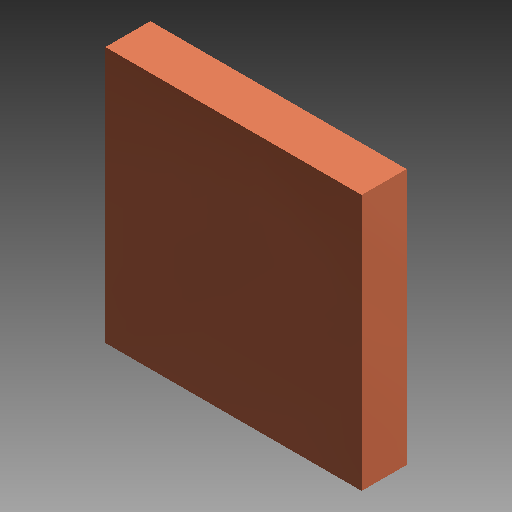
# Autodesk Inventor part: Atmega32u2
Saved by Autodesk Inventor 2018.2 (Build 222227000, 227)
## iProperties
Part Number: Atmega32u2
Material: Generic
Document SubType Name: Modeling
Designer: autocad
Appearance: QFN32_050050, Atmega32u2
Author: autocad
Autodesk Inventor part; units mm, degrees
ref_plane "YZ Plane" through (0, 0, 0) normal (1, 0, 0) x (0, 1, 0)
ref_plane "XZ Plane" through (0, 0, 0) normal (0, 1, 0) x (-1, 0, 0)
ref_plane "XY Plane" through (0, 0, 0) normal (0, 0, 1) x (1, 0, 0)
sketch "QFN32_050050, Atmega32u2_285" plane through (0, 0, 0) normal (0, 0, 1) x (1, 0, 0)
  line L0 (-2.8405, -2.8405) -> (-2.8405, 2.8575)
  line L1 (-2.8405, 2.8575) -> (2.8575, 2.8575)
  line L2 (2.8575, 2.8575) -> (2.8575, -2.8405)
  line L3 (2.8575, -2.8405) -> (-2.8405, -2.8405)
  constraints: 8 end point
extrude "Extrusion1" add sketch "QFN32_050050, Atmega32u2_285" along normal blind 1
body "Solid1"
